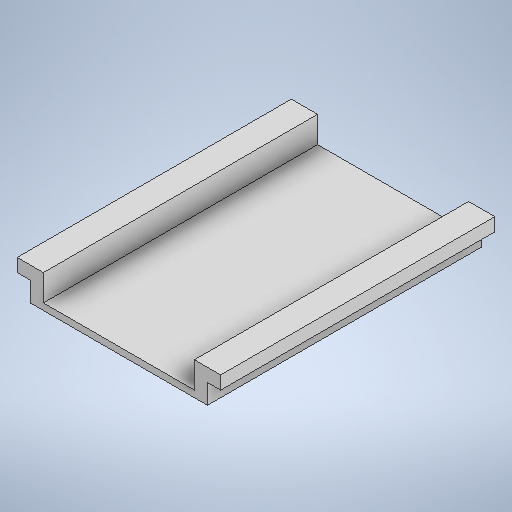
# Autodesk Inventor part: Avionics Cradle (12-13)
Saved by Autodesk Inventor 2025.2 (Build 292293000, 293)
## iProperties
Created: 2025-01-28
Part Number: Avionics Cradle (12-13)
Material: Generic
Document SubType Name: Modeling
Designer: Tia
Density: 1 g/cm^3
Appearance: Default
Author: Tia
Autodesk Inventor part; units mm, degrees
ref_plane "YZ Plane" through (0, 0, 0) normal (1, 0, 0) x (0, 1, 0)
ref_plane "XZ Plane" through (0, 0, 0) normal (0, 1, 0) x (-1, 0, 0)
ref_plane "XY Plane" through (0, 0, 0) normal (0, 0, 1) x (1, 0, 0)
sketch "Sketch2" plane through (0, 0, 0) normal (0, 0, 1) x (1, 0, 0)
  line L0 (-14.9328, -5.3201) -> (-10.9328, -5.3201)
  line L1 (-10.9328, -5.3201) -> (-10.9328, -11.3201)
  line L2 (-10.9328, -11.3201) -> (20.0672, -11.3201)
  line L3 (-10.9328, -11.3201) -> (20.0672, -11.3201)
  line L4 (20.0672, -11.3201) -> (20.0672, -9.3157)
  line L5 (20.0672, -9.3157) -> (-6.9328, -9.3157)
  line L6 (-6.9328, -9.3157) -> (-6.9328, -1.3157)
  line L7 (-6.9328, -1.3157) -> (-14.9328, -1.3157)
  line L8 (-14.9328, -1.3157) -> (-14.9328, -5.3157)
  line L9 (-14.9328, -5.3157) -> (-10.9328, -5.3157)
  line L10 (-14.9328, -1.3157) -> (-6.9328, -1.3157)
  line L11 (-6.9328, -1.3157) -> (-6.9328, -9.3157)
  line L12 (-6.9328, -9.3157) -> (16.0672, -9.3157)
  line L13 (16.0672, -9.3157) -> (16.0672, -11.3157)
  line L14 (16.0672, -11.3157) -> (-10.9328, -11.3201)
  line L15 (-10.9328, -11.3201) -> (-10.9328, -5.3157)
  line L16 (-10.9328, -5.3157) -> (-14.9328, -5.3157)
  line L17 (-14.9328, -1.3157) -> (-14.9328, -5.3157)
  point P0 (0, 0)
  point P1 (-14.9328, 16.2146)
  point P2 (20.0672, -10.3179)
  point P3 (-12.9328, -5.3201)
  dimension "d0" = 27
  dimension "d1" = 8
  dimension "d2" = 8
  dimension "d3" = 90
  dimension "d4" = 4
  dimension "d5" = 90
  dimension "d6" = 4
  dimension "d7" = 90
  dimension "d8" = 23
  dimension "d9" = 2
  constraints: 36 end point, 11 perpendicular, 2 midpoint, 1 horizontal, 1 parallel, 1 point on line, 1 vertical, 2 other
  measures "d0" distance of L4.end L5.end
  measures "d1" distance of L5.end L6.end
  measures "d2" distance of L6.end L7.end
  measures "d3" angle of L7 L6
  measures "d4" distance of L7.end L8.end
  measures "d5" angle of L8 L7
  measures "d6" distance of L8.end L9.end
  measures "d7" angle of L9 L8
  measures "d8" distance of L5.end L12.end
  measures "d9" distance of L12.end L13.end
extrude "Extrusion1" add sketch "Sketch2" along normal blind 83.525 contours L15 L9 L8 L7 L6 L5 L13 L14 L1
mirror "Mirror1" about plane through (16.0672, -11.3157, 0) normal (1, 0, 0) of "Extrusion1"
body "Solid1"
